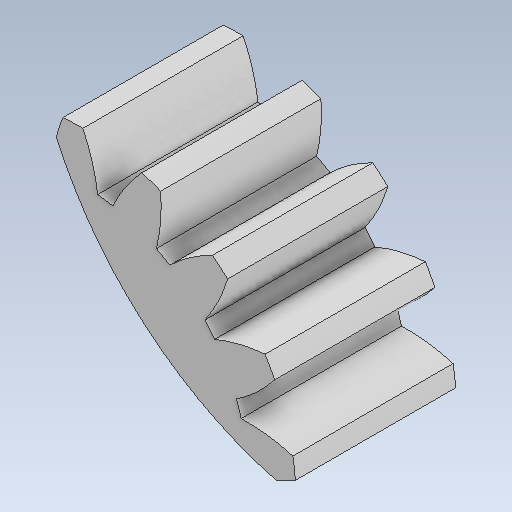
# Autodesk Inventor part: small-gear
Saved by Autodesk Inventor 2020 (Build 240168000, 168)
## iProperties
Created: 2020-05-22
Part Number: small-gear
Material: Ogólny
Document SubType Name: Modeling
Designer: blep
Density: 1 g/cm^3
Appearance: Domyślna
Author: blep
Autodesk Inventor part; units mm, degrees
ref_plane "YZ Plane" through (0, 0, 0) normal (1, 0, 0) x (0, 1, 0)
ref_plane "XZ Plane" through (0, 0, 0) normal (0, 1, 0) x (-1, 0, 0)
ref_plane "XY Plane" through (0, 0, 0) normal (0, 0, 1) x (1, 0, 0)
sketch "Szkic1" plane through (0, 0, 0) normal (0, 0, 1) x (1, 0, 0)
  arc A0 (-1.732, -4.0613) -> (-1.6613, -4.132) centre (0, -2.4) ccw projected
  arc A1 (0.05, -0.4006) -> (-0.05, -0.4006) centre (0, -2.4) ccw projected
  arc A2 (-0.05, -0.4006) -> (-0.5703, -0.483) centre (0, -2.4) ccw projected
  arc A3 (-0.5703, -0.483) -> (-0.6654, -0.5139) centre (0, -2.4) ccw projected
  arc A4 (-0.6654, -0.5139) -> (-1.1348, -0.7531) centre (0, -2.4) ccw projected
  arc A5 (-1.1348, -0.7531) -> (-1.2157, -0.8119) centre (0, -2.4) ccw projected
  arc A6 (-1.2157, -0.8119) -> (-1.5881, -1.1843) centre (0, -2.4) ccw projected
  arc A7 (-1.5881, -1.1843) -> (-1.6469, -1.2652) centre (0, -2.4) ccw projected
  arc A8 (-1.6469, -1.2652) -> (-1.8861, -1.7346) centre (0, -2.4) ccw projected
  arc A9 (-1.8861, -1.7346) -> (-1.917, -1.8297) centre (0, -2.4) ccw projected
  arc A10 (-1.917, -1.8297) -> (-1.9994, -2.35) centre (0, -2.4) ccw projected
  arc A11 (-1.9994, -2.35) -> (-1.9994, -2.45) centre (0, -2.4) ccw projected
  arc A12 (-1.9994, -2.45) -> (-1.917, -2.9703) centre (0, -2.4) ccw projected
  arc A13 (-1.917, -2.9703) -> (-1.8861, -3.0654) centre (0, -2.4) ccw projected
  arc A14 (-1.8861, -3.0654) -> (-1.6469, -3.5348) centre (0, -2.4) ccw projected
  arc A15 (-1.6469, -3.5348) -> (-1.5881, -3.6157) centre (0, -2.4) ccw projected
  arc A16 (-1.5881, -3.6157) -> (-1.2157, -3.9881) centre (0, -2.4) ccw projected
  arc A17 (-1.2157, -3.9881) -> (-1.1348, -4.0469) centre (0, -2.4) ccw projected
  arc A18 (-1.1348, -4.0469) -> (-0.6654, -4.2861) centre (0, -2.4) ccw projected
  arc A19 (-0.6654, -4.2861) -> (-0.5703, -4.317) centre (0, -2.4) ccw projected
  arc A20 (-0.5703, -4.317) -> (-0.05, -4.3994) centre (0, -2.4) ccw projected
  arc A21 (-0.05, -4.3994) -> (0.05, -4.3994) centre (0, -2.4) ccw projected
  arc A22 (0.05, -4.3994) -> (0.5703, -4.317) centre (0, -2.4) ccw projected
  arc A23 (0.5703, -4.317) -> (0.6654, -4.2861) centre (0, -2.4) ccw projected
  arc A24 (0.6654, -4.2861) -> (1.1348, -4.0469) centre (0, -2.4) ccw projected
  arc A25 (1.1348, -4.0469) -> (1.2157, -3.9881) centre (0, -2.4) ccw projected
  arc A26 (1.2157, -3.9881) -> (1.5881, -3.6157) centre (0, -2.4) ccw projected
  arc A27 (1.5881, -3.6157) -> (1.6469, -3.5348) centre (0, -2.4) ccw projected
  arc A28 (1.6469, -3.5348) -> (1.8861, -3.0654) centre (0, -2.4) ccw projected
  arc A29 (1.8861, -3.0654) -> (1.917, -2.9703) centre (0, -2.4) ccw projected
  arc A30 (1.917, -2.9703) -> (1.9994, -2.45) centre (0, -2.4) ccw projected
  arc A31 (1.9994, -2.45) -> (1.9994, -2.35) centre (0, -2.4) ccw projected
  arc A32 (1.9994, -2.35) -> (1.917, -1.8297) centre (0, -2.4) ccw projected
  arc A33 (1.917, -1.8297) -> (1.8861, -1.7346) centre (0, -2.4) ccw projected
  arc A34 (1.8861, -1.7346) -> (1.6469, -1.2652) centre (0, -2.4) ccw projected
  arc A35 (1.6469, -1.2652) -> (1.5881, -1.1843) centre (0, -2.4) ccw projected
  arc A36 (1.5881, -1.1843) -> (1.2157, -0.8119) centre (0, -2.4) ccw projected
  arc A37 (1.2157, -0.8119) -> (1.1348, -0.7531) centre (0, -2.4) ccw projected
  arc A38 (1.1348, -0.7531) -> (0.6654, -0.5139) centre (0, -2.4) ccw projected
  arc A39 (0.6654, -0.5139) -> (0.5703, -0.483) centre (0, -2.4) ccw projected
  arc A40 (0.5703, -0.483) -> (0.05, -0.4006) centre (0, -2.4) ccw projected
  circle A41 centre (0, -2.4) radius 1.5065 projected
  circle A42 centre (0, -2.4) radius 2.4
  circle A43 centre (0, -2.4) radius 15
  circle A44 centre (0, -2.4) radius 1.0065 projected
  circle A45 centre (0, -2.4) radius 1.2565
  circle A46 centre (0, -2.4) radius 2.9
  point P0 (0, 0)
  point P1 (-1.6613, -4.132)
  point P2 (-1.732, -4.0613)
  dimension "d0" = 30
  dimension "d3" = 0.25
  dimension "d12" = 0.5
  constraints: 4 centre point, 2 coincident, 1 concentric
  measures "d0" diameter of A43
  measures "d3" radial gap between concentric circles of A44 A45
  measures "d12" radial gap between concentric circles of A42 A46
extrude "Wyciągnięcie proste1" add sketch "Szkic1" against normal blind 3 contours A43
extrude "Wyciągnięcie proste2" add sketch "Szkic1" along normal blind 1.5 contours A42 A0 | A40 A39 A38 A37 A36 A35 A34 A33 A32 A31 A30 A29 A28 A27 A26 A25 A24 A23 A22 A21 A20 A19 A18 A17 A16 A15 A14 A13 A12 A11 A10 A9 A8 A7 A6 A5 A4 A3 A2 A1 | A41 | A43 | A45 | A46
sketch "Szkic2" plane through (0, -2.4, 1.5) normal (0, 0, 1) x (1, 0, 0)
  circle A0 centre (0, 0) radius 1.0065 projected
  circle A1 centre (0, 0) radius 3
  circle A2 centre (0, 0) radius 15 projected
  point P0 (0, 2.4)
  dimension "d6" = 6
  constraints: 1 centre point, 1 coincident
  measures "d6" diameter of A1
extrude "Wyciągnięcie proste3" add sketch "Szkic2" along normal blind 2.7 contours A2
sketch "Szkic4" plane through (0, -2.4, -3) normal (0, 0, -1) x (-1, 0, 0)
  arc A0 (6.703, -7.1797) -> (6.021, -7.7605) centre (12.6436, -14.8459) ccw projected
  arc A1 (9.8735, -5.5514) -> (9.0277, -5.8466) centre (12.6436, -14.8459) ccw projected
  arc A2 (13.4181, -5.1783) -> (12.5228, -5.1481) centre (12.6436, -14.8459) ccw projected
  arc A3 (16.8582, -6.1109) -> (16.0342, -5.7593) centre (12.6436, -14.8459) ccw projected
  arc A4 (19.729, -8.2232) -> (19.0877, -7.5977) centre (12.6436, -14.8459) ccw projected
  arc A5 (21.6429, -11.23) -> (21.2709, -10.4151) centre (12.6436, -14.8459) ccw projected
  arc A6 (22.3415, -14.7251) -> (22.2889, -13.8308) centre (12.6436, -14.8459) ccw projected
  arc A7 (21.7302, -18.2365) -> (22.0043, -17.3836) centre (12.6436, -14.8459) ccw projected
  arc A8 (19.8918, -21.29) -> (20.4555, -20.5937) centre (12.6436, -14.8459) ccw projected
  arc A9 (3.9087, -10.6314) -> (5.6223, -12.2259) centre (9.734, -6.0892) ccw projected
  arc A10 (5.6223, -12.2259) -> (5.4105, -12.8849) centre (12.6436, -14.8459) ccw projected
  arc A11 (5.4105, -12.8849) -> (3.0888, -13.1827) centre (5.1774, -20.2681) ccw projected
  arc A12 (3.0888, -13.1827) -> (2.9761, -14.0714) centre (12.6436, -14.8459) ccw projected
  arc A13 (2.9761, -14.0714) -> (5.1499, -14.9393) centre (6.7672, -7.7316) ccw projected
  arc A14 (5.1499, -14.9393) -> (5.1905, -15.6303) centre (12.6436, -14.8459) ccw projected
  arc A15 (5.1905, -15.6303) -> (3.1332, -16.7466) centre (7.6403, -22.5991) ccw projected
  arc A16 (3.1332, -16.7466) -> (3.3491, -17.616) centre (12.6436, -14.8459) ccw projected
  arc A17 (3.3491, -17.616) -> (5.6897, -17.64) centre (4.594, -10.3348) ccw projected
  arc A18 (5.6897, -17.64) -> (5.9772, -18.2697) centre (12.6436, -14.8459) ccw projected
  arc A19 (5.9772, -18.2697) -> (4.462, -20.0539) centre (10.7789, -23.883) ccw projected
  arc A20 (4.462, -20.0539) -> (4.9774, -20.7866) centre (12.6436, -14.8459) ccw projected
  arc A21 (4.9774, -20.7866) -> (7.1686, -19.9634) centre (3.508, -13.5473) ccw projected
  arc A22 (7.1686, -19.9634) -> (7.6642, -20.4467) centre (12.6436, -14.8459) ccw projected
  arc A23 (7.6642, -20.4467) -> (6.8958, -22.6577) centre (14.1694, -23.9463) ccw projected
  arc A24 (6.8958, -22.6577) -> (7.6411, -23.1547) centre (12.6436, -14.8459) ccw projected
  arc A25 (7.6411, -23.1547) -> (9.387, -21.5956) centre (3.6558, -16.9352) ccw projected
  arc A26 (9.387, -21.5956) -> (10.0237, -21.8673) centre (12.6436, -14.8459) ccw projected
  arc A27 (10.0237, -21.8673) -> (10.1059, -24.2066) centre (17.3539, -22.7806) ccw projected
  arc A28 (10.1059, -24.2066) -> (10.9804, -24.4008) centre (12.6436, -14.8459) ccw projected
  arc A29 (10.9804, -24.4008) -> (12.0452, -22.3162) centre (5.0175, -20.0409) ccw projected
  arc A30 (12.0452, -22.3162) -> (12.737, -22.3396) centre (12.6436, -14.8459) ccw projected
  arc A31 (12.737, -22.3396) -> (13.6588, -24.4912) centre (19.9021, -20.5433) ccw projected
  arc A32 (13.6588, -24.4912) -> (14.5444, -24.3564) centre (12.6436, -14.8459) ccw projected
  arc A33 (14.5444, -24.3564) -> (14.7842, -22.028) centre (7.4091, -22.4449) ccw projected
  arc A34 (14.7842, -22.028) -> (15.4377, -21.7998) centre (12.6436, -14.8459) ccw projected
  arc A35 (15.4377, -21.7998) -> (17.0745, -23.4732) centre (21.4701, -17.5365) ccw projected
  arc A36 (17.0745, -23.4732) -> (17.8516, -23.0275) centre (12.6436, -14.8459) ccw projected
  arc A37 (17.8516, -23.0275) -> (17.2341, -20.7697) centre (10.5077, -23.8227) ccw projected
  arc A38 (17.2341, -20.7697) -> (17.7611, -20.3209) centre (12.6436, -14.8459) ccw projected
  arc A39 (17.7611, -20.3209) -> (19.8918, -21.29) centre (21.846, -14.1663) ccw projected
  arc A40 (20.4555, -20.5937) -> (19.0641, -18.7114) centre (13.8947, -23.9881) ccw projected
  arc A41 (19.0641, -18.7114) -> (19.3933, -18.1026) centre (12.6436, -14.8459) ccw projected
  arc A42 (19.3933, -18.1026) -> (21.7302, -18.2365) centre (20.9791, -10.8879) ccw projected
  arc A43 (22.0043, -17.3836) -> (20.0269, -16.1311) centre (17.1128, -22.9188) ccw projected
  arc A44 (20.0269, -16.1311) -> (20.114, -15.4444) centre (12.6436, -14.8459) ccw projected
  arc A45 (20.114, -15.4444) -> (22.3415, -14.7251) centre (18.9865, -8.1441) ccw projected
  arc A46 (22.2889, -13.8308) -> (19.9926, -13.3772) centre (19.7273, -20.7593) ccw projected
  arc A47 (19.9926, -13.3772) -> (19.8257, -12.7054) centre (12.6436, -14.8459) ccw projected
  arc A48 (19.8257, -12.7054) -> (21.6429, -11.23) centre (16.1372, -6.3053) ccw projected
  arc A49 (21.2709, -10.4151) -> (18.9658, -10.8216) centre (21.3851, -17.801) ccw projected
  arc A50 (18.9658, -10.8216) -> (18.5675, -10.2554) centre (12.6436, -14.8459) ccw projected
  arc A51 (18.5675, -10.2554) -> (19.729, -8.2232) centre (12.816, -5.6201) ccw projected
  arc A52 (19.0877, -7.5977) -> (17.0851, -8.8095) centre (21.8623, -14.4437) ccw projected
  arc A53 (17.0851, -8.8095) -> (16.5092, -8.4255) centre (12.6436, -14.8459) ccw projected
  arc A54 (16.5092, -8.4255) -> (16.8582, -6.1109) centre (9.4716, -6.1808) ccw projected
  arc A55 (16.0342, -5.7593) -> (14.6046, -7.6127) centre (21.0945, -11.1407) ccw projected
  arc A56 (14.6046, -7.6127) -> (13.9288, -7.4626) centre (12.6436, -14.8459) ccw projected
  arc A57 (13.9288, -7.4626) -> (13.4181, -5.1783) centre (6.5556, -7.9118) ccw projected
  arc A58 (12.5228, -5.1481) -> (11.8593, -7.3928) centre (19.1854, -8.3381) ccw projected
  arc A59 (11.8593, -7.3928) -> (11.1749, -7.4969) centre (12.6436, -14.8459) ccw projected
  arc A60 (11.1749, -7.4969) -> (9.8735, -5.5514) centre (4.4619, -10.5793) ccw projected
  arc A61 (9.0277, -5.8466) -> (9.2198, -8.1794) centre (16.3927, -6.4144) ccw projected
  arc A62 (9.2198, -8.1794) -> (8.6193, -8.5238) centre (12.6436, -14.8459) ccw projected
  arc A63 (8.6193, -8.5238) -> (6.703, -7.1797) centre (3.4731, -13.823) ccw projected
  arc A64 (6.021, -7.7605) -> (7.0428, -9.8664) centre (13.0938, -5.6294) ccw projected
  arc A65 (7.0428, -9.8664) -> (6.6073, -10.4044) centre (12.6436, -14.8459) ccw projected
  arc A66 (6.6073, -10.4044) -> (4.3348, -9.8434) centre (3.7228, -17.2049) ccw projected
  arc A67 (4.3348, -9.8434) -> (3.9087, -10.6314) centre (12.6436, -14.8459) ccw projected
  point P0 (0, 2.4)
  point P1 (0, 0)
extrude "Wyciągnięcie proste5" cut sketch "Szkic4" against normal blind 10 keep common part
